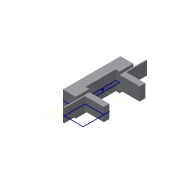
# Autodesk Inventor part: 17-0028-0085
Saved by Autodesk Inventor 2016 SP2 (Build 200236200, 236)
## iProperties
Category: IOP
Company: Universiteit van Amsterdam
Created: 2017-11-24
Part Number: 17-0028-0085
Material: Generic
Document SubType Name: Modeling
Designer: Daan Giesen
Density: 1 g/cm^3
Appearance: Default
Project: Digital PID Loop
Cost Center: 17-0028
User Status: Work in Progress
Authority: Reichsöllner, Lukas
Author: Daan Giesen
Title: Digital PID Loop
Revision Number: A
Autodesk Inventor part; units mm, degrees
ref_plane "YZ Plane" through (0, 0, 0) normal (1, 0, 0) x (0, 1, 0)
ref_plane "XZ Plane" through (0, 0, 0) normal (0, 1, 0) x (-1, 0, 0)
ref_plane "XY Plane" through (0, 0, 0) normal (0, 0, 1) x (1, 0, 0)
sketch "Sketch1" plane through (0, 0, 0) normal (0, 0, 1) x (1, 0, 0)
  line L0 (0, 113.8) -> (0, -147.3) construction
  line L1 (-34.4, 0) -> (87.4, 0) construction
  line L2 (-17, 76.5) -> (17, 76.5)
  line L3 (17, 76.5) -> (17, -76.5)
  line L4 (17, -76.5) -> (-17, -76.5)
  line L5 (-17, -76.5) -> (-17, 76.5)
  line L6 (-17, 76.5) -> (17, -76.5) construction
  line L7 (17, 76.5) -> (-17, -76.5) construction
  line L8 (7, 40) -> (17, 40)
  line L9 (17, 40) -> (17, -40)
  line L10 (17, -40) -> (7, -40)
  line L11 (7, -40) -> (7, 40)
  line L12 (7, 40) -> (17, -40) construction
  line L13 (17, 40) -> (7, -40) construction
  line L14 (17, -40) -> (70, -40)
  line L15 (70, -40) -> (70, -110)
  line L16 (70, -110) -> (17, -110)
  line L17 (17, -110) -> (17, -40)
  line L18 (70, -110) -> (20, -110)
  line L19 (20, -110) -> (20, -55)
  line L20 (20, -55) -> (70, -55)
  line L21 (70, -55) -> (70, -110)
  point P0 (0, 0)
  point P1 (12, 0)
  dimension "d4" = 80
  dimension "d5" = 153
  dimension "d6" = 34
  dimension "d7" = 10
  dimension "d10" = 70
  dimension "d11" = 55
  dimension "d12" = 53
  dimension "d13" = 3
  constraints: 40 end point, 8 parallel, 4 horizontal, 4 midpoint, 4 perpendicular, 2 point on line
  measures "d4" distance of L10.end L8.start
  measures "d5" distance of L4.end L2.start
  measures "d6" distance of L3.end L4.end
  measures "d7" distance of L9.end L10.end
  measures "d10" distance of L16.end L9.end
  measures "d11" distance of L18.end L19.end
  measures "d12" distance of L9.end L14.end
  measures "d13" distance between parallel lines of L3 L19
extrude "Extrusion3" add sketch "Sketch1" along normal mid plane 50 contours L2 L3 L8 L11 L10 L4 L5
extrude "Extrusion4" add sketch "Sketch1" along normal mid plane 35 contours L3 L14 L15 L20 L19 L16 L17
mirror "Mirror1" about plane through (0, 0, 0) normal (0, 1, 0) of "Extrusion4"
body "Solid3"
